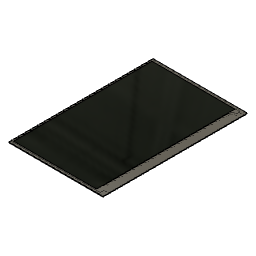
Updated_OpenBookEnclosure2v16 (Autodesk Fusion 360 archive; units mm, degrees)
design "DisplayEbook"
Autodesk Fusion 360 part; units mm, degrees
sketch "Sketch1" plane through (0, 0, 0) normal (0, 0, 1) x (1, 0, 0)
  line L0 (-60, 75) -> (51.2, 75)
  line L1 (51.2, 75) -> (51.2, -95.2)
  line L2 (51.2, -95.2) -> (-60, -95.2)
  line L3 (-60, -95.2) -> (-60, 75)
  dimension "d1" = 111.2
  dimension "d2" = 170.2
  constraint horizontal L0
  constraint vertical L1
  constraint horizontal L2
  constraint vertical L3
  measures "d1" distance of L0.start L0.end
  measures "d2" distance of L0.start L2.end
extrude "Extrude1" add sketch "Sketch1" along normal blind 0.2 makes body 1
sketch "Sketch2" plane through (0, 0, 0.2) normal (0, 0, 1) x (-1, 0, 0)
  line L0 (60, 95.2) -> (-51.2, 95.2)
  line L1 (-51.2, 95.2) -> (-51.2, -75)
  line L2 (-51.2, -75) -> (60, -75)
  line L3 (60, -75) -> (60, 95.2)
  line L4 (-48.8868, 93.9459, 0.2) -> (58.2032, 93.9459, 0.2)
  line L5 (58.2032, 93.9459, 0.2) -> (58.2032, -73.8541, 0.2)
  line L6 (58.2032, -73.8541, 0.2) -> (-48.8868, -73.8541, 0.2)
  line L7 (-48.8868, -73.8541, 0.2) -> (-48.8868, 93.9459, 0.2)
  line L8 (-55.1941, 80.895, 0.1772) -> (-55.1941, -60, 0.2102)
  arc A0 through (-55.1941, -60, 0.2102) (-48.8868, -66.3073, 0.2015) (-42.5795, -60, 0.1898)
  line L9 (-42.5795, -60, 0.1898) -> (-42.5795, 80.895, 0.1567)
  arc A1 through (-42.5795, 80.895, 0.1567) (-48.8868, 87.2023, 0.1655) (-55.1941, 80.895, 0.1772)
  line L10 (-48.8868, 80.895, 0.167) -> (-48.8868, -60, 0.2) construction
  dimension "d5" = 107.09
  dimension "d6" = 167.8
extrude "Extrude2" add sketch "Sketch2" along normal blind 0.2 contours L4 L5 L6 L7 in plane through (0, 0, 0.4) normal (0, 0, 1) bodies 1 makes body 2
sketch "Sketch3" plane through (0, 0, 0.6) normal (0, 0, 1) x (-1, 0, 0)
  line L0 (-48.8868, -73.8541) -> (58.2032, -73.8541)
  line L1 (58.2032, -73.8541) -> (58.2032, 93.9459)
  line L2 (58.2032, 93.9459) -> (-48.8868, 93.9459)
  line L3 (-48.8868, 93.9459) -> (-48.8868, -73.8541)
  line L4 (-45.1811, 92.4092) -> (58.9089, 92.4092)
  line L5 (58.9089, 92.4092) -> (58.9089, -72.3908)
  line L6 (58.9089, -72.3908) -> (-45.1811, -72.3908)
  line L7 (-45.1811, -72.3908) -> (-45.1811, 92.4092)
  line L8 (-50.1811, 82.6471) -> (-50.1811, -63.4885)
  arc A0 (-50.1811, -63.4885) -> (-40.1811, -63.4885) centre (-45.1811, -63.4885) ccw
  line L9 (-40.1811, -63.4885) -> (-40.1811, 82.6471)
  arc A1 (-40.1811, 82.6471) -> (-50.1811, 82.6471) centre (-45.1811, 82.6471) ccw
  line L10 (-45.1811, 82.6471) -> (-45.1811, -63.4885) construction
  dimension "d9" = 104.09
  dimension "d10" = 164.8
  dimension "d14" = 10
  constraint horizontal L4
  constraint vertical L5
  constraint horizontal L6
  constraint vertical L7
  constraint tangent L8 A0
  constraint tangent A0 L9
  constraint parallel L8 L9
  constraint tangent L9 A1
  constraint tangent L8 A1
  constraint coincident L7 A0.centre
  constraint parallel L3 L10
  measures "d9" distance of L4.start L4.end
  measures "d10" distance of L4.start L6.end
  measures "d14" diameter of A0
move_face "MoveFace1" by (-1.4, 0, 0) 2 faces at (-58.2032, -38.0126, 0.4667) (48.8868, 17.9207, 0.4667) on bodies 2
extrude "Extrude3" add sketch "Sketch3" along normal blind 0.4 contours L1 L4 L6 L7 A0 L9 A1 bodies 1 2
sketch "Sketch4" plane through (0, 0, 0.6) normal (0, 0, 1) x (-1, 0, 0)
  line L0 (58.2032, -72.3908) -> (-45.1811, -72.3908)
  line L1 (-45.1811, -72.3908) -> (-45.1811, -68.4885)
  arc A0 (-45.1811, -68.4885) -> (-40.1811, -63.4885) centre (-45.1811, -63.4885) ccw
  line L2 (-40.1811, -63.4885) -> (-40.1811, 82.6471)
  arc A1 (-40.1811, 82.6471) -> (-45.1811, 87.6471) centre (-45.1811, 82.6471) ccw
  line L3 (-45.1811, 87.6471) -> (-45.1811, 92.4092)
  line L4 (-45.1811, 92.4092) -> (58.2032, 92.4092)
  line L5 (58.2032, 92.4092) -> (58.2032, -72.3908)
  line L6 (-47.4868, -73.8541) -> (59.6032, -73.8541)
  line L7 (59.6032, -73.8541) -> (59.6032, 93.9459)
  line L8 (59.6032, 93.9459) -> (-47.4868, 93.9459)
  line L9 (-47.4868, 93.9459) -> (-47.4868, -73.8541)
  line L10 (-41.5379, -60.6884) -> (-41.5379, 79.1866)
  arc A2 (-41.5379, 79.1866) -> (-53.4356, 79.1866) centre (-47.4868, 79.1866) ccw
  line L11 (-53.4356, 79.1866) -> (-53.4356, -60.6884)
  arc A3 (-53.4356, -60.6884) -> (-41.5379, -60.6884) centre (-47.4868, -60.6884) ccw
  line L12 (-47.4868, -60.6884) -> (-47.4868, 79.1866) construction
  constraint tangent L10 A2
  constraint tangent A2 L11
  constraint parallel L10 L11
  constraint tangent L11 A3
  constraint tangent L10 A3
  constraint coincident L9 A2.centre
  constraint coincident L9 A3.centre
extrude "Extrude4" cut sketch "Sketch4" against normal blind 0.2 contours L9 L10 A2 A3 bodies 2
sketch "Sketch5" plane through (0, 0, 1) normal (0, 0, 1) x (-1, 0, 0)
  line L0 (58.2032, -72.3908) -> (58.2032, 92.4092)
  line L1 (58.2032, 92.4092) -> (-45.1811, 92.4092)
  line L2 (-45.1811, 92.4092) -> (-45.1811, 87.6471)
  arc A0 (-40.1811, 82.6471) -> (-45.1811, 87.6471) centre (-45.1811, 82.6471) ccw
  line L3 (-40.1811, 82.6471) -> (-40.1811, -63.4885)
  arc A1 (-45.1811, -68.4885) -> (-40.1811, -63.4885) centre (-45.1811, -63.4885) ccw
  line L4 (-45.1811, -68.4885) -> (-45.1811, -72.3908)
  line L5 (-45.1811, -72.3908) -> (58.2032, -72.3908)
  line L6 (-39.8749, 91.5282, 0.1) -> (58.0451, 91.5282, 0.1)
  line L7 (58.0451, 91.5282, 0.1) -> (58.0451, -71.6718, 0.1)
  line L8 (58.0451, -71.6718, 0.1) -> (-39.8749, -71.6718, 0.1)
  line L9 (-39.8749, -71.6718, 0.1) -> (-39.8749, 91.5282, 0.1)
  dimension "d19" = 97.92
  dimension "d20" = 163.2
move_body "Move1" bodies 1 to x (1, 0, 0) y (0, 1, 0) z (0, 0, 1) at (0, 0, 1)
move_face "MoveFace2" by (0, 0, 0.5) 1 faces at (-22.9333, 18.2667, 1.2) on bodies 1
sketch "Sketch6" plane through (0, 0, 1.1) normal (0, 0, 1) x (-1, 0, 0)
move_body "Move2" bodies 1 2 to x (1, 0, 0) y (0, 1, 0) z (0, 0, 1) at (0, 0, -0.4)
sketch "Sketch7" plane through (0, 0, 0) normal (0, 1, 0) x (1, 0, 0)
move_face "MoveFace3" by (0, 0, -0.2) 1 faces at (-25.4085, -34.2218, 0.6) on bodies 2
move_body "Move3" bodies 1 to x (1, 0, 0) y (0, 1, 0) z (0, 0, 1) at (0, 0, -0.2)
extrude "Extrude6" add sketch "Sketch5" along normal blind 0.08 contours L6 L7 L8 L9 in plane through (0, 0, 1.1) normal (0, 0, 1) bodies 1

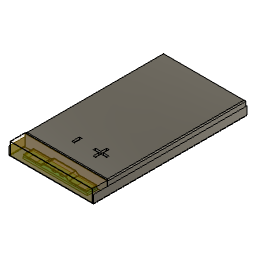
design "Battery"
Autodesk Fusion 360 part; units mm, degrees
sketch "Sketch1" plane through (0, 0, 0) normal (0, 0, 1) x (1, 0, 0)
  line L0 (20, -40) -> (-21.3329, -40)
  line L1 (-21.3329, -40) -> (-21.3329, 34.7664)
  line L2 (-21.3329, 34.7664) -> (20, 34.7664)
  line L3 (20, 34.7664) -> (20, -40)
  constraint horizontal L0
  constraint vertical L1
  constraint horizontal L2
  constraint vertical L3
sketch "Sketch2" plane through (0, 0, 0) normal (0, 0, 1) x (1, 0, 0)
  line L0 (-22, 34.5) -> (19, 34.5)
  line L1 (19, 34.5) -> (19, -34.35)
  line L2 (19, -34.35) -> (-22, -34.35)
  line L3 (-22, -34.35) -> (-22, 34.5)
  dimension "d3" = 68.85
  dimension "d30" = 41
  constraint horizontal L0
  constraint vertical L1
  constraint horizontal L2
  constraint vertical L3
  measures "d3" distance of L0.start L2.end
  measures "d30" distance of L0.start L0.end
extrude "Extrude2" add sketch "Sketch2" along normal blind 6.2 makes body 1
move_body "Move1" bodies 1 to x (1, 0, 0) y (0, -1, 0) z (0, 0, -1) at (0, 0.05, 0)
sketch "Sketch3" plane through (0, 0, -6.2) normal (0, 0, -1) x (1, 0, 0)
  line L0 (-22, -34.4) -> (19, -34.4)
  line L1 (19, -34.4) -> (19, 34.45)
  line L2 (19, 34.45) -> (-22, 34.45)
  line L3 (-22, 34.45) -> (-22, -34.4)
sketch "Sketch4" plane through (0, 0, 0) normal (0, 0, 1) x (1, 0, 0)
  line L0 (-22.5409, 34.3667) -> (19.4591, 34.3667)
  line L1 (19.4591, 34.3667) -> (19.4591, -42.1333)
  line L2 (19.4591, -42.1333) -> (-22.5409, -42.1333)
  line L3 (-22.5409, -42.1333) -> (-22.5409, 34.3667)
  dimension "d7" = 76.5
  dimension "d31" = 42
  constraint horizontal L0
  constraint vertical L1
  constraint horizontal L2
  constraint vertical L3
  measures "d7" distance of L0.start L2.end
  measures "d31" distance of L1.end L2.end
move_body "Move2" bodies 1 to x (1, 0, 0) y (0, 1, 0) z (0, 0, 1) at (0, 0, 6.25)
surface "Extrude3" add extruded along (0, 0, 1) between 0 and 4 profiles "Sketch4" section 1 separate body makes body 2
move_body "Move3" bodies 2 to x (1, 0, 0) y (0, 1, 0) z (0, 0, 1) at (0, 0.2, 0)
sketch "Sketch5" plane through (0, 0, 0.05) normal (0, 0, -1) x (1, 0, 0)
  line L0 (-22, -34.4) -> (19, -34.4)
  line L1 (19, -34.4) -> (19, 34.45)
  line L2 (19, 34.45) -> (-22, 34.45)
  line L3 (-22, 34.45) -> (-22, -34.4)
  line L4 (-22.555, -34.5709) -> (19.445, -34.5709)
  line L5 (19.445, -34.5709) -> (19.445, 41.9096)
  line L6 (19.445, 41.9096) -> (-22.555, 41.9096)
  line L7 (-22.555, 41.9096) -> (-22.555, -34.5709)
  dimension "d32" = 42
  constraint horizontal L4
  constraint vertical L5
  constraint horizontal L6
  constraint vertical L7
  measures "d32" distance of L5.end L6.end
extrude "Extrude4" add sketch "Sketch5" along normal blind 0.2 separate body makes body 3
delete_face "SurfaceDeleteFace1" leaving the opening 1 faces at (5.4591, -41.9333, 1.3333) on bodies 2
delete_face "SurfaceDeleteFace2" leaving the opening 1 faces at (-8.5409, 34.5667, 1.3333) on bodies 2 makes body 4 at (19.4591, 9.0667, 1.3333)
fillet "Fillet1" radius 0.5 tangency weight 2 4 edges at (-1.5, -34.45, 6.25) (19, -0.025, 6.25) (-22, -0.025, 6.25) (-1.5, 34.4, 6.25) on bodies 1
sketch "Sketch7" plane through (0, 0, 6.25) normal (0, 0, 1) x (-1, 0, 0)
  line L0 (21.5, -33.9) -> (-18.5, -33.9)
  line L1 (21.5, 33.95) -> (21.5, -33.9)
  line L2 (-18.5, 33.95) -> (21.5, 33.95)
  line L3 (-18.5, -33.9) -> (-18.5, 33.95)
  line L4 (-2.3447, 29.7125) -> (-17, 29.7125) construction
  line L5 (-17, 29.7125) -> (-17, 21) construction
  line L6 (-17, 21) -> (-2.3447, 21) construction
  line L7 (-2.3447, 21) -> (-2.3447, 29.7125) construction
  line L8 (10.6965, 22.8914) -> (10.6318, 29.6721) construction
  line L9 (10.6318, 29.6721) -> (5.2715, 29.621) construction
  line L10 (5.2715, 29.621) -> (5.3361, 22.8402) construction
  line L11 (5.3361, 22.8402) -> (10.6965, 22.8914) construction
  dimension "d17" = 10
  dimension "d18" = 10
  text T0 "+" font "Arial" height 10 align left top in box 14.6553 x 8.7125 at (-2.3447, 29.7125) x (-1, 0) y (0, -1) spacing 1 kerned
  text T1 "-" font "Arial" height 10 align left top in box 6.781 x 5.3606 at (10.6965, 22.8914) x (-0.009537, 0.999955) y (-0.999955, -0.009537) spacing 1 kerned
extrude "Extrude5" cut sketch "Sketch7" against normal blind 1 text T0 T1 bodies 1
sketch "Sketch8" plane through (0, 0, 0) normal (0, 0, 1) x (1, 0, 0)
  line L0 (-20, -43) -> (20, -43)
  line L1 (20, -43) -> (20, -48)
  line L2 (20, -48) -> (-20, -48)
  line L3 (-20, -48) -> (-20, -43)
  constraint horizontal L0
  constraint vertical L1
  constraint horizontal L2
  constraint vertical L3
extrude "Extrude6" add sketch "Sketch8" along normal blind 1 separate body makes body 5
move_body "Move4" bodies 5 to x (1, 0, 0) y (0, 1, 0) z (0, 0, 1) at (0, 8, 1)
sketch "Sketch9" plane through (0, 0, 2) normal (0, 0, 1) x (-1, 0, 0)
  line L0 (20, 40) -> (-20, 40)
  line L1 (-20, 40) -> (-20, 35)
  line L2 (-20, 35) -> (20, 35)
  line L3 (20, 35) -> (20, 40)
  line L4 (-14, 37) -> (-10, 37)
  line L5 (-10, 37) -> (-10, 40)
  line L6 (-10, 40) -> (-14, 40)
  line L7 (-14, 40) -> (-14, 37)
  constraint horizontal L4
  constraint vertical L5
  constraint horizontal L6
  constraint vertical L7
extrude "Extrude7" add sketch "Sketch9" along normal blind 0.1 contours L0 L4 L5 L6 L7 bodies 5
sketch "Sketch10" plane through (0, 0, 2) normal (0, 0, 1) x (-1, 0, 0)
  line L0 (-10, 40) -> (-10, 37)
  line L1 (-10, 37) -> (-14, 37)
  line L2 (-14, 37) -> (-14, 40)
  line L3 (-14, 40) -> (-20, 40)
  line L4 (-20, 40) -> (-20, 35)
  line L5 (-20, 35) -> (20, 35)
  line L6 (20, 35) -> (20, 40)
  line L7 (20, 40) -> (-10, 40)
  line L8 (14, 37) -> (10, 37)
  line L9 (10, 37) -> (10, 40)
  line L10 (10, 40) -> (14, 40)
  line L11 (14, 40) -> (14, 37)
  constraint horizontal L8
  constraint vertical L9
  constraint horizontal L10
  constraint vertical L11
  constraint coincident L7 L9.end
extrude "Extrude8" add sketch "Sketch10" along normal blind 0.1 contours L7 L8 L9 L10 L11 bodies 5
sketch "Sketch11" plane through (0, 0, 2) normal (0, 0, 1) x (-1, 0, 0)
  line L0 (10, 37) -> (10, 40)
  line L1 (10, 40) -> (-10, 40)
  line L2 (-10, 40) -> (-10, 37)
  line L3 (-10, 37) -> (-14, 37)
  line L4 (-14, 37) -> (-14, 40)
  line L5 (-14, 40) -> (-20, 40)
  line L6 (-20, 40) -> (-20, 35)
  line L7 (-20, 35) -> (20, 35)
  line L8 (20, 35) -> (20, 40)
  line L9 (20, 40) -> (14, 40)
  line L10 (14, 40) -> (14, 37)
  line L11 (14, 37) -> (10, 37)
  line L12 (3, 37) -> (1, 37)
  line L13 (1, 37) -> (1, 39)
  line L14 (1, 39) -> (3, 39)
  line L15 (3, 39) -> (3, 37)
  line L16 (-1, 37) -> (-3, 37)
  line L17 (-3, 37) -> (-3, 39)
  line L18 (-3, 39) -> (-1, 39)
  line L19 (-1, 39) -> (-1, 37)
  constraint horizontal L12
  constraint vertical L13
  constraint horizontal L14
  constraint vertical L15
  constraint horizontal L16
  constraint vertical L17
  constraint horizontal L18
  constraint vertical L19
extrude "Extrude9" add sketch "Sketch11" along normal blind 0.1 contours L12 L13 L14 L15 | L16 L17 L18 L19 bodies 5
move_face "MoveFace1" by (-4, 0, 0) 1 faces at (20, -36.6667, 1.3333) on bodies 5
move_face "MoveFace2" by (4, 0, 0) 1 faces at (-20, -38.3333, 1.3333) on bodies 5
move_body "Move5" bodies 5 to x (1, 0, 0) y (0, 1, 0) z (0, 0, 1) at (0, 0, -1)
sketch "Sketch12" plane through (0, 0, 0.05) normal (0, 0, 1) x (-1, 0, 0)
  line L0 (-19, 34.45) -> (22, 34.45)
  line L1 (22.555, -34.5709) -> (22.555, 41.9096)
  line L2 (22.555, 41.9096) -> (-19.445, 41.9096)
  line L3 (-19.445, 41.9096) -> (-19.445, -34.5709)
  line L4 (-19.445, -34.5709) -> (22.555, -34.5709)
  line L5 (22, -34.4) -> (-19, -34.4)
  line L6 (-19, -34.4) -> (-19, 34.45)
  line L7 (22, 34.45) -> (22, -34.4)
move_body "Move6" bodies 5 to x (1, 0, 0) y (0, 1, 0) z (0, 0, 1) at (-1.5, 0, 0)
sketch "Sketch13" plane through (0, 0, 0) normal (0, 0, 1) x (1, 0, 0)
sketch "Sketch14" plane through (0, 0, 0) normal (1, 0, 0) x (0, 1, 0)
  line L0 (-40, 6) -> (-35, 6)
  line L1 (-35, 6) -> (-35, 5.5979)
  line L2 (-35, 5.5979) -> (-40, 5.5979)
  line L3 (-40, 5.5979) -> (-40, 6)
  dimension "d41" = 5
  constraint horizontal L0
  constraint vertical L1
  constraint horizontal L2
  constraint vertical L3
  measures "d41" distance of L1.end L2.end
sketch "Sketch15" plane through (0, 0, 0) normal (0, 1, 0) x (1, 0, 0)
  line L0 (-8, -9) -> (4.3629, -9)
  line L1 (4.3629, -9) -> (6, -8)
  line L2 (6, -8) -> (12, -8)
  line L3 (-8, -9) -> (-9.6419, -8.0065)
  line L4 (-9.6419, -8.0065) -> (-15.3019, -8.0065)
  constraint horizontal L0
  constraint parallel L0 L2
  constraint parallel L0 L4
sweep "Sweep1" add profiles "Sketch14" path "Sketch15" along L4 L3 L0 L1 L2 section 1 separate body makes body 6
move_body "Move7" bodies 6 to x (1, 0, 0) y (0, 1, 0) z (0, 0, 1) at (0.25, 0, -3)
move_body "Move8" bodies 6 to x (1, 0, 0) y (0, 1, 0) z (0, 0, 1) at (0, 2, 0)
move_body "Move9" bodies 6 to x (1, 0, 0) y (0, 1, 0) z (0, 0, 1) at (0, -1.5, 0)
move_body "Move10" bodies 6 to x (1, 0, 0) y (0, 1, 0) z (0, 0, 1) at (0, -0.5, 0)
move_face "MoveFace3" by (2, 0, 0) 1 faces at (12.25, -38.3333, 1.7319) on bodies 6
move_face "MoveFace4" by (-2.2, 0, 0) 1 faces at (-15.0519, -36.6667, 1.8725) on bodies 6
sketch "Sketch16" plane through (0, 0, 0) normal (0, 1, 0) x (1, 0, 0)
  line L0 (-23, -7) -> (-23, -13.3)
  line L1 (-23, -13.3) -> (19, -13.3)
  line L2 (19, -13.3) -> (19, -7)
  dimension "d42" = 6.3
  constraint vertical L0
  constraint perpendicular L0 L1
  constraint perpendicular L1 L2
  measures "d42" distance of L0.start L0.end
sketch "Sketch17" plane through (0, 0, 0) normal (1, 0, 0) x (0, 1, 0)
  line L0 (-41.8993, 7.3012) -> (-34.5, 7.3012)
  line L1 (-34.5, 7.3012) -> (-34.5, 7.2012)
  line L2 (-34.5, 7.2012) -> (-41.8993, 7.2012)
  line L3 (-41.8993, 7.2012) -> (-41.8993, 7.3012)
  dimension "d43" = 0.1
  constraint horizontal L0
  constraint vertical L1
  constraint horizontal L2
  constraint vertical L3
  measures "d43" distance of L0.start L2.end
sweep "Sweep2" add profiles "Sketch17" path "Sketch16" along L0 L1 L2 section 1 separate body makes body 7
move_face "MoveFace5" by (6, 0, 0) 2 faces at (12.9012, -36.9664, 7.1341) (13.0012, -36.9664, 7.1004) on bodies 7
move_face "MoveFace6" by (-5, 0, 0) 2 faces at (-17.0012, -39.4329, 7.1004) (-16.9012, -39.4329, 7.1341) on bodies 7
move_body "Move11" bodies 7 to x (1, 0, 0) y (0, 1, 0) z (0, 0, 1) at (0, 0, -1.1)
move_face "MoveFace7" by (0, 0, -5.8) 2 faces at (18.9679, -36.9664, 5.9) (-21.9679, -36.9664, 5.9) on bodies 7
sketch "Sketch18" plane through (0, -41.8993, 0) normal (0, -1, 0) x (1, 0, 0)
  line L0 (-21.9012, 6.1012) -> (18.9012, 6.1012)
  line L1 (18.9012, 6.1012) -> (18.9012, 0.1)
  line L2 (18.9012, 0.1) -> (19.0012, 0.1)
  line L3 (19.0012, 0.1) -> (19.0012, 6.2012)
  line L4 (19.0012, 6.2012) -> (-22.0012, 6.2012)
  line L5 (-22.0012, 6.2012) -> (-22.0012, 0.1)
  line L6 (-22.0012, 0.1) -> (-21.9012, 0.1)
  line L7 (-21.9012, 0.1) -> (-21.9012, 6.1012)
  line L8 (-22.0012, 6.2012) -> (19.0012, 6.2012)
  line L9 (19.0012, 6.2012) -> (19.0012, 0.1)
  line L10 (19.0012, 0.1) -> (-22.0012, 0.1)
  line L11 (-22.0012, 0.1) -> (-22.0012, 6.2012)
  line L12 (-22.0012, 6.2012) -> (19.0012, 6.2012)
  line L13 (19.0012, 6.2012) -> (19.0012, 0.1)
  line L14 (19.0012, 0.1) -> (-22.0012, 0.1)
  line L15 (-22.0012, 0.1) -> (-22.0012, 6.2012)
  constraint horizontal L8
  constraint vertical L9
  constraint horizontal L10
  constraint vertical L11
  constraint coincident L2.end L3.start
  constraint coincident L4.end L5.start
  constraint horizontal L12
  constraint vertical L13
  constraint horizontal L14
  constraint vertical L15
extrude "Extrude10" add sketch "Sketch18" along normal blind 0.1 contours L0 L1 L7 L10 L14 bodies 7
